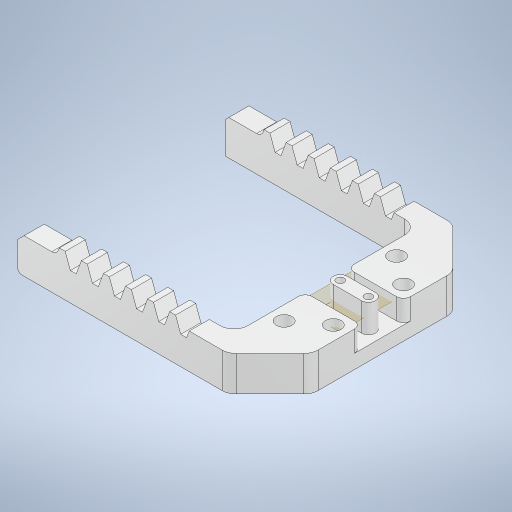
# Autodesk Inventor part: Rack
Saved by Autodesk Inventor 2023.4 (Build 274418000, 418)
## iProperties
Created: 2024-01-11
Part Number: Rack
Material: Aluminum 6061
Document SubType Name: Modeling
Designer: Nathan Cai
Mass: 18.3268 g
Surface Area: 57.6486 cm^2
Volume: 6.78771 cm^3
Density: 2.7 g/cm^3
Appearance: Aluminum - Flat
Author: Nathan Cai
Autodesk Inventor part; units mm, degrees
ref_plane "YZ Plane" through (0, 0, 0) normal (1, 0, 0) x (0, 1, 0)
ref_plane "XZ Plane" through (0, 0, 0) normal (0, 1, 0) x (-1, 0, 0)
ref_plane "XY Plane" through (0, 0, 0) normal (0, 0, 1) x (1, 0, 0)
sketch "Sketch1" plane through (0, 0, 0) normal (0, 1, 0) x (-1, 0, 0)
  line L0 (22.225, 20.85) -> (-22.225, 20.85)
  line L1 (-22.225, 20.85) -> (-22.225, -20.85)
  line L2 (-22.225, -20.85) -> (22.225, -20.85)
  line L3 (22.225, -20.85) -> (22.225, 20.85)
  line L4 (22.225, 20.85) -> (-22.225, -20.85) construction
  line L5 (-22.225, 20.85) -> (22.225, -20.85) construction
  line L6 (0, 0) -> (-22.225, 0) construction
  line L7 (22.225, 25.4) -> (-34.925, 25.4)
  line L8 (-34.925, 25.4) -> (-34.925, -25.4)
  line L9 (-34.925, -25.4) -> (22.225, -25.4)
  line L10 (22.225, -25.4) -> (22.225, 25.4)
  line L11 (22.225, 25.4) -> (-34.925, -25.4) construction
  line L12 (-34.925, 25.4) -> (22.225, -25.4) construction
  point P0 (-6.35, 0)
  point P1 (22.225, 20.85)
  dimension "d0" = 44.45
  dimension "d1" = 41.7
  dimension "d3" = 12.7
  dimension "d198" = 50.8
  constraints: 26 end point, 5 midpoint, 4 parallel, 2 horizontal, 2 perpendicular, 2 point on line
  measures "d0" distance of L2.end L1.end
  measures "d1" distance of L1.end L0.end
  measures "d3" distance between parallel lines of L1 L8
  measures "d198" distance between parallel lines of L7 L9
extrude "Extrusion1" add sketch "Sketch1" along normal blind 9.525 contours L0 L1 L2 L10 L9 L8 L7
chamfer "Chamfer1" distance 9.525 angle 45 2 edges at (34.925, 4.7625, 25.4) (34.925, 4.7625, -25.4)
fillet "Fillet1" radius 3.175 4 edges at (25.4, 4.7625, -25.4) (34.925, 4.7625, -15.875) (34.925, 4.7625, 15.875) (25.4, 4.7625, 25.4)
fillet "Fillet4" radius 3.175 2 edges at (22.225, 4.7625, -20.85) (22.225, 4.7625, 20.85)
sketch "Sketch5" plane through (-22.225, 0, -25.4) normal (0, 0, -1) x (-1, 0, 0)
  line L0 (0, 0) -> (0, 9.525) projected
  line L1 (0, 9.525) -> (-46.3099, 9.525) projected
  line L2 (-10.8754, 9.525) -> (-12.031, 6.35)
  line L3 (-12.031, 6.35) -> (-13.369, 6.35)
  line L4 (-13.369, 6.35) -> (-14.5246, 9.525)
  line L5 (-25.4, 9.525) -> (-25.4, 6.35) construction
  line L6 (0, 9.525) -> (0, 6.35) construction
  line L7 (-12.7, 9.525) -> (-12.7, 6.35) construction
  line L8 (-25.4, 7.9375) -> (0, 7.9375) construction
  line L9 (-15.8627, 9.525) -> (-17.0183, 6.35)
  line L10 (-17.0183, 6.35) -> (-18.3563, 6.35)
  line L11 (-18.3563, 6.35) -> (-19.5119, 9.525)
  line L12 (-17.6873, 9.525) -> (-17.6873, 6.35) construction
  line L13 (-20.8499, 9.525) -> (-22.0055, 6.35)
  line L14 (-22.0055, 6.35) -> (-23.3436, 6.35)
  line L15 (-23.3436, 6.35) -> (-24.4992, 9.525)
  line L16 (-22.6746, 9.525) -> (-22.6746, 6.35) construction
  line L17 (-25.8372, 9.525) -> (-26.9928, 6.35)
  line L18 (-26.9928, 6.35) -> (-28.3309, 6.35)
  line L19 (-28.3309, 6.35) -> (-29.4865, 9.525)
  line L20 (-27.6618, 9.525) -> (-27.6618, 6.35) construction
  line L21 (-30.8245, 9.525) -> (-31.9801, 6.35)
  line L22 (-31.9801, 6.35) -> (-33.3181, 6.35)
  line L23 (-33.3181, 6.35) -> (-34.4737, 9.525)
  line L24 (-32.6491, 9.525) -> (-32.6491, 6.35) construction
  line L25 (-35.8118, 9.525) -> (-36.9674, 6.35)
  line L26 (-36.9674, 6.35) -> (-38.3054, 6.35)
  line L27 (-38.3054, 6.35) -> (-39.461, 9.525)
  line L28 (-37.6364, 9.525) -> (-37.6364, 6.35) construction
  line L29 (-12.031, 6.35) -> (0, 6.35)
  line L30 (-5.8881, 9.525) -> (-7.0437, 6.35)
  line L31 (-8.3817, 6.35) -> (-9.5373, 9.525)
  line L32 (-8.9595, 7.9375) -> (0, 7.9375)
  arc A0 (-8.3817, 6.35) -> (-7.0437, 6.35) centre (-7.7127, 6.5935) ccw
  arc A1 (-13.369, 6.35) -> (-12.031, 6.35) centre (-12.7, 6.5935) ccw
  arc A2 (-18.3563, 6.35) -> (-17.0183, 6.35) centre (-17.6873, 6.5935) ccw
  arc A3 (-23.3436, 6.35) -> (-22.0055, 6.35) centre (-22.6746, 6.5935) ccw
  arc A4 (-28.3309, 6.35) -> (-26.9928, 6.35) centre (-27.6618, 6.5935) ccw
  arc A5 (-33.3181, 6.35) -> (-31.9801, 6.35) centre (-32.6491, 6.5935) ccw
  arc A6 (-38.3054, 6.35) -> (-36.9674, 6.35) centre (-37.6364, 6.5935) ccw
  point P0 (-22.225, 0)
  point P1 (-13.9468, 7.9375)
  point P2 (-11.4532, 7.9375)
  point P3 (-11.4532, 7.9375)
  point P4 (-16.4405, 7.9375)
  point P5 (-16.4405, 7.9375)
  point P6 (-4.9873, 6.35)
  point P7 (-30.3873, 6.35)
  point P8 (-18.9341, 7.9375)
  point P9 (-21.4277, 7.9375)
  point P10 (-21.4277, 7.9375)
  point P11 (-9.9746, 6.35)
  point P12 (-35.3746, 6.35)
  point P13 (-23.9214, 7.9375)
  point P14 (-26.415, 7.9375)
  point P15 (-26.415, 7.9375)
  point P16 (-14.9618, 6.35)
  point P17 (-40.3618, 6.35)
  point P18 (-28.9087, 7.9375)
  point P19 (-31.4023, 7.9375)
  point P20 (-31.4023, 7.9375)
  point P21 (-19.9491, 6.35)
  point P22 (-45.3491, 6.35)
  point P23 (-33.8959, 7.9375)
  point P24 (-36.3896, 7.9375)
  point P25 (-36.3896, 7.9375)
  point P26 (-24.9364, 6.35)
  point P27 (-50.3364, 6.35)
  point P28 (-38.8832, 7.9375)
  point P29 (-24.4992, 9.525)
  point P30 (-6.4659, 7.9375)
  point P31 (-6.4659, 7.9375)
  point P32 (0, 7.9375)
  dimension "d68" = 3.175
  dimension "d70" = 70
  dimension "d71" = 2.4936
  dimension "d74" = 4.9873
  dimension "d79" = 12.7
  dimension "d82" = 4.9873
  dimension "d175" = 4.9873
  constraints: 62 end point, 20 point on line, 18 midpoint, 14 point on circle, 7 centre point, 5 horizontal, 2 tangent, 1 collinear, 1 vertical, 110 other
  measures "d68" distance from line of L1 L6.end
  measures "d70" angle of L3 L2
  measures "d71" distance of point (-11.453, 7.938) point (-13.947, 7.938)
  measures "d74" distance of L2.start L9.start
  measures "d79" distance between parallel lines of L0 L7
  measures "d82" distance of L2.start L30.start
  measures "d175" distance of A0.centre A1.centre
extrude "Extrusion8" cut sketch "Sketch5" against normal through all contours L32 L30 L1 L0 | L32 L31 L1 L30 | L3 L4 L1 L2 | L9 L10 L11 L1 | L13 L14 L15 L1 | L17 L18 L19 L1 | L21 L22 L23 L1 | L25 L26 L27 L1
fillet "Fillet5" radius 1.5875 2 edges at (-13.2655, 7.9375, -23.125) (-13.2655, 7.9375, 23.125)
chamfer "Chamfer3" distance 1.5875 angle 45 2 edges at (-22.225, 7.9375, -23.125) (-22.225, 7.9375, 23.125)
chamfer "Chamfer4" distance 0.7937 angle 45 2 edges at (-22.225, 0, -23.125) (-22.225, 0, 23.125)
sketch "Sketch8" plane through (0, 9.525, 0) normal (0, 1, 0) x (1, 0, 0)
  line L0 (22.225, 17.675) -> (22.225, -17.675) projected
  line L1 (22.225, 0) -> (34.925, 0) construction
  line L2 (34.925, -14.5599) -> (34.925, 14.5599) projected
  line L3 (28.575, 0) -> (22.225, 0) construction
  line L4 (25.4, -7.9375) -> (31.75, -7.9375) construction
  line L5 (31.75, -7.9375) -> (31.75, 7.9375) construction
  line L6 (31.75, 7.9375) -> (25.4, 7.9375) construction
  line L7 (25.4, 7.9375) -> (25.4, -7.9375) construction
  line L8 (25.4, -7.9375) -> (31.75, 7.9375) construction
  line L9 (31.75, -7.9375) -> (25.4, 7.9375) construction
  circle A0 centre (25.4, 7.9375) radius 1.7526
  circle A1 centre (31.75, 7.9375) radius 1.7526
  circle A2 centre (25.4, -7.9375) radius 1.7526
  circle A3 centre (31.75, -7.9375) radius 1.7526
  circle A4 centre (25.4, 12.7) radius 1.7526
  circle A5 centre (25.4, -12.7) radius 1.7526
  circle A6 centre (34.925, 0) radius 4.7625
  line L10 (9.525, 0) -> (34.925, 0) construction
  line L11 (9.525, -4.7625) -> (34.925, -4.7625)
  line L12 (34.925, 4.7625) -> (9.525, 4.7625)
  arc A7 (9.525, 4.7625) -> (9.525, -4.7625) centre (9.525, 0) ccw
  arc A8 (34.925, -4.7625) -> (34.925, 4.7625) centre (34.925, 0) ccw
  line L13 (31.75, 0) -> (25.4, 0) construction
  line L14 (31.75, 1.5875) -> (25.4, 1.5875)
  line L15 (25.4, -1.5875) -> (31.75, -1.5875)
  arc A9 (31.75, -1.5875) -> (31.75, 1.5875) centre (31.75, 0) ccw
  arc A10 (25.4, 1.5875) -> (25.4, -1.5875) centre (25.4, 0) ccw
  circle A11 centre (25.4, 0) radius 0.875
  circle A12 centre (31.75, 0) radius 0.875
  point P0 (0, 0)
  point P1 (22.225, -4.7625)
  point P2 (22.225, 4.7625)
  point P3 (34.925, 4.7625)
  point P4 (34.925, -4.7625)
  dimension "d122" = 6.35
  dimension "d123" = 15.875
  dimension "d124" = 3.5052
  dimension "d127" = 6.35
  dimension "d130" = 15.875
  dimension "d136" = 3.5052
  dimension "d137" = 12.7
  dimension "d172" = 9.525
  dimension "d186" = 9.525
  dimension "d190" = 3.175
  dimension "d191" = 1.75
  dimension "d192" = 1.75
  constraints: 34 end point, 13 centre point, 9 midpoint, 8 point on circle, 8 tangent, 4 parallel, 3 coincident, 3 collinear, 2 horizontal, 1 perpendicular, 1 point on line, 1 symmetric about line, 1 vertical, 7 other
  measures "d122" distance of L6.end L5.end
  measures "d123" distance of L5.end L4.end
  measures "d124" diameter of A0
  measures "d127" distance of A0.centre A1.centre
  measures "d130" distance of A0.centre A2.centre
  measures "d136" diameter of A4
  measures "d137" distance from line of L3 A4.centre
  measures "d172" diameter of A6
  measures "d186" distance between parallel lines of L11 L12
  measures "d190" diameter of A10
  measures "d191" diameter of A11
  measures "d192" diameter of A12
extrude "Extrusion11" cut sketch "Sketch8" against normal through all contours A1 | A3 | A4 | A5
extrude "Extrusion12" cut sketch "Sketch8" against normal blind 6.35 contours L12 A6 L14 A10 L15 L11 L0 | L0 L11 A7 L12 | A6 L2 | L2 A6 L15 A9 L14
fillet "Fillet6" radius 1.5875 4 edges at (22.225, 6.35, 4.7625) (22.225, 6.35, -4.7625) (34.925, 6.35, 4.7625) (34.925, 6.35, -4.7625)
fillet "Fillet8" [suppressed]
ref_plane "Work Plane2" through (0, 6.35, 0) normal (0, 1, 0) x (1, 0, 0)
chamfer "Chamfer8" distance 0.7937 angle 45 2 edges at (-22.225, 3.5719, -20.85) (-22.225, 3.5719, 20.85)
sketch "Sketch13" plane through (0, 9.525, 0) normal (0, 1, 0) x (1, 0, 0)
  line L0 (34.925, 6.35) -> (34.925, 14.5599) projected
  arc A0 (34.925, 14.5599) -> (33.9951, 16.8049) centre (31.75, 14.5599) ccw projected
  line L1 (26.3299, 24.4701) -> (33.9951, 16.8049) projected
  arc A1 (26.3299, 24.4701) -> (24.0849, 25.4) centre (24.0849, 22.225) ccw projected
  line L2 (24.0849, 25.4) -> (17.236, 25.4) projected
  line L3 (17.236, 25.4) -> (17.236, 20.85) projected
  line L4 (17.236, 20.85) -> (19.05, 20.85) projected
  arc A2 (22.225, 17.675) -> (19.05, 20.85) centre (19.05, 17.675) ccw projected
  line L5 (22.225, 17.675) -> (22.225, 6.35) projected
  line L6 (23.8125, 4.7625) -> (33.3375, 4.7625) projected
  circle A3 centre (25.4, 12.7) radius 1.7526 projected
  circle A4 centre (31.75, 7.9375) radius 1.7526 projected
  circle A5 centre (25.4, -12.7) radius 1.7526 projected
  circle A6 centre (31.75, -7.9375) radius 1.7526 projected
  line L7 (33.3375, -4.7625) -> (23.8125, -4.7625) projected
  line L8 (22.225, -6.35) -> (22.225, -17.675) projected
  arc A7 (19.05, -20.85) -> (22.225, -17.675) centre (19.05, -17.675) ccw projected
  line L9 (19.05, -20.85) -> (17.236, -20.85) projected
  line L10 (17.236, -20.85) -> (17.236, -25.4) projected
  line L11 (17.236, -25.4) -> (24.0849, -25.4) projected
  arc A8 (24.0849, -25.4) -> (26.3299, -24.4701) centre (24.0849, -22.225) ccw projected
  line L12 (33.9951, -16.8049) -> (26.3299, -24.4701) projected
  arc A9 (33.9951, -16.8049) -> (34.925, -14.5599) centre (31.75, -14.5599) ccw projected
  line L13 (34.925, -14.5599) -> (34.925, -6.35) projected
  line L14 (17.236, 20.85) -> (16.0804, 20.85) projected
  line L15 (17.236, 25.4) -> (17.236, 20.85) projected
  line L16 (16.0804, 25.4) -> (17.236, 25.4) projected
  line L17 (16.0804, 25.4) -> (16.0804, 20.85) projected
  line L18 (16.0804, -20.85) -> (17.236, -20.85) projected
  line L19 (16.0804, -20.85) -> (16.0804, -25.4) projected
  line L20 (17.236, -25.4) -> (16.0804, -25.4) projected
  line L21 (17.236, -20.85) -> (17.236, -25.4) projected
  line L22 (23.8125, 4.7625) -> (33.3375, 4.7625) projected
  line L23 (34.925, 6.35) -> (34.925, 14.5599) projected
  arc A10 (34.925, 14.5599) -> (33.9951, 16.8049) centre (31.75, 14.5599) ccw projected
  line L24 (26.3299, 24.4701) -> (33.9951, 16.8049) projected
  arc A11 (26.3299, 24.4701) -> (24.0849, 25.4) centre (24.0849, 22.225) ccw projected
  line L25 (24.0849, 25.4) -> (17.236, 25.4) projected
  line L26 (17.236, 25.4) -> (17.236, 20.85) projected
  line L27 (17.236, 20.85) -> (19.05, 20.85) projected
  arc A12 (22.225, 17.675) -> (19.05, 20.85) centre (19.05, 17.675) ccw projected
  line L28 (22.225, 17.675) -> (22.225, 6.35) projected
  line L29 (33.3375, -4.7625) -> (23.8125, -4.7625) projected
  line L30 (22.225, -6.35) -> (22.225, -17.675) projected
  arc A13 (19.05, -20.85) -> (22.225, -17.675) centre (19.05, -17.675) ccw projected
  line L31 (19.05, -20.85) -> (17.236, -20.85) projected
  line L32 (17.236, -20.85) -> (17.236, -25.4) projected
  line L33 (17.236, -25.4) -> (24.0849, -25.4) projected
  arc A14 (24.0849, -25.4) -> (26.3299, -24.4701) centre (24.0849, -22.225) ccw projected
  line L34 (33.9951, -16.8049) -> (26.3299, -24.4701) projected
  arc A15 (33.9951, -16.8049) -> (34.925, -14.5599) centre (31.75, -14.5599) ccw projected
  line L35 (34.925, -14.5599) -> (34.925, -6.35) projected
  arc A16 (33.3375, 4.7625) -> (34.925, 6.35) centre (33.3375, 6.35) ccw projected
  arc A17 (22.225, 6.35) -> (23.8125, 4.7625) centre (23.8125, 6.35) ccw projected
  arc A18 (34.925, -6.35) -> (33.3375, -4.7625) centre (33.3375, -6.35) ccw projected
  arc A19 (23.8125, -4.7625) -> (22.225, -6.35) centre (23.8125, -6.35) ccw projected
  arc A20 (33.3375, 4.7625) -> (34.925, 6.35) centre (33.3375, 6.35) ccw projected
  arc A21 (22.225, 6.35) -> (23.8125, 4.7625) centre (23.8125, 6.35) ccw projected
  arc A22 (34.925, -6.35) -> (33.3375, -4.7625) centre (33.3375, -6.35) ccw projected
  arc A23 (23.8125, -4.7625) -> (22.225, -6.35) centre (23.8125, -6.35) ccw projected
  point P0 (0, 0)
  point P1 (17.236, 25.4)
  point P2 (17.236, -25.4)
  point P3 (17.236, 25.4)
  point P4 (17.236, -25.4)
extrude "Extrusion17" cut sketch "Sketch13" against normal blind 1.5875 contours A16 L6 A17 L5 A2 L4 L3 L2 A1 L1 A0 L0 | L3 L14 L17 L16 | A3 | A4 | A5 | A6 | A18 L13 A9 L12 A8 L11 L10 L9 A7 L8 A19 L7 | L10 L20 L19 L18
extrude "Extrusion18" cut sketch "Sketch8" against normal blind 3.175 contours A11 | A12
equation "\"d71\" = 0.5 * d69"
equation "\"d74\" = 1.5708 * d68"
equation "\"d82\" = d74"
equation "\"d127\" = d122"
equation "\"d130\" = d123"
equation "\"d69\" = 1.5708 * d68"
body "Solid1"
